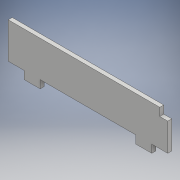
# Autodesk Inventor part: ramp-support
Saved by Autodesk Inventor 2017 (Build 210142000, 142)
## iProperties
Created: 2017-03-05
Part Number: ramp-support
Material: Generic
Document SubType Name: Modeling
Designer: John
Density: 1 g/cm^3
Appearance: Default
Author: John
Autodesk Inventor part; units mm, degrees
ref_plane "YZ Plane" through (0, 0, 0) normal (1, 0, 0) x (0, 1, 0)
ref_plane "XZ Plane" through (0, 0, 0) normal (0, 1, 0) x (-1, 0, 0)
ref_plane "XY Plane" through (0, 0, 0) normal (0, 0, 1) x (1, 0, 0)
sketch "Sketch1" plane through (0, 0, 0) normal (0, 1, 0) x (-1, 0, 0)
  line L0 (0, 0) -> (120, 0)
  line L1 (120, 0) -> (120, 27)
  line L2 (120, 27) -> (0, 27)
  line L3 (0, 27) -> (0, 0)
  dimension "d5" = 120
  dimension "d6" = 27
  constraints: 8 end point, 2 perpendicular, 1 horizontal, 1 vertical
  measures "d5" distance of L0.start L0.end
  measures "d6" distance of L0.end L1.end
extrude "Extrusion1" add sketch "Sketch1" along normal blind 3
sketch "Sketch2" plane through (0, 0, 0) normal (0, -1, 0) x (1, 0, 0)
  line L0 (-120, 27) -> (0, 27) projected
  line L1 (0, 27) -> (-6, 27)
  line L2 (-6, 27) -> (-6, 21)
  line L3 (-6, 21) -> (0, 21)
  line L4 (0, 21) -> (0, 27)
  point P0 (0, 0)
  dimension "d7" = 6
  dimension "d8" = 6
  constraints: 8 end point, 2 parallel, 1 horizontal, 1 perpendicular
  measures "d7" distance of L3.end L2.end
  measures "d8" distance of L2.end L1.end
extrude "Extrusion2" cut sketch "Sketch2" along normal through all both and the other way through all
sketch "Sketch3" plane through (0, 0, 0) normal (0, -1, 0) x (1, 0, 0)
  line L0 (0, 0) -> (-120, 0) projected
  line L1 (-108, 0) -> (-96, 0)
  line L2 (-96, 0) -> (-96, -6)
  line L3 (-96, -6) -> (-108, -6)
  line L4 (-108, -6) -> (-108, 0)
  line L5 (-12, 0) -> (-24, 0)
  line L6 (-24, 0) -> (-24, -6)
  line L7 (-24, -6) -> (-12, -6)
  line L8 (-12, -6) -> (-12, 0)
  line L9 (0, 21) -> (0, 0) projected
  line L10 (-120, 0) -> (-120, 27) projected
  dimension "d11" = 12
  dimension "d12" = 6
  dimension "d13" = 12
  dimension "d14" = 6
  dimension "d15" = 12
  dimension "d16" = 12
  constraints: 16 end point, 4 parallel, 2 horizontal, 2 perpendicular, 2 point on line
  measures "d11" distance of L2.end L3.end
  measures "d12" distance of L1.end L2.end
  measures "d13" distance of L7.end L6.end
  measures "d14" distance of L6.end L5.end
  measures "d15" distance between parallel lines of L9 L8
  measures "d16" distance between parallel lines of L4 L10
extrude "Extrusion3" add sketch "Sketch3" against normal blind 3
body "Solid1"
